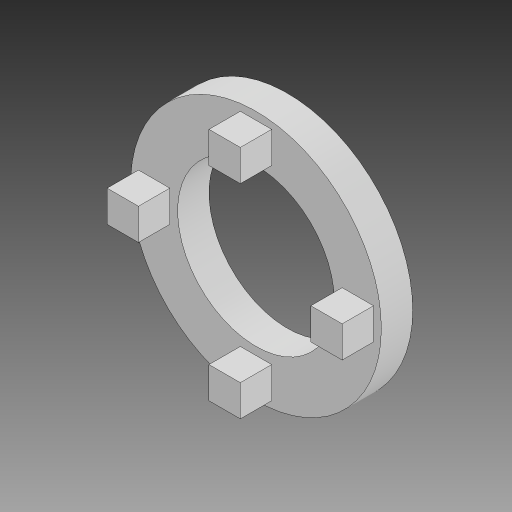
# Autodesk Inventor part: support-ring
Saved by Autodesk Inventor 2023 (Build 270158000, 158)
## iProperties
Created: 2024-01-30
Part Number: support-ring
Material: Všeobecné
Document SubType Name: Modeling
Designer: matej
Mass: 0.0346305 g
Surface Area: 1.18102 cm^2
Volume: 0.0346305 cm^3
Density: 1 g/cm^3
Appearance: Výchozí
Author: matej
Autodesk Inventor part; units mm, degrees
ref_plane "YZ Plane" through (0, 0, 0) normal (1, 0, 0) x (0, 1, 0)
ref_plane "XZ Plane" through (0, 0, 0) normal (0, 1, 0) x (-1, 0, 0)
ref_plane "XY Plane" through (0, 0, 0) normal (0, 0, 1) x (1, 0, 0)
sketch "Náčrt1" plane through (0, 0, 0) normal (0, 0, 1) x (1, 0, 0)
  circle A0 centre (0, 0) radius 2.5
  circle A1 centre (0, 0) radius 4
  dimension "d0" = 5
  dimension "d1" = 8
  constraints: 2 centre point, 2 coincident
  measures "d0" diameter of A0
  measures "d1" diameter of A1
extrude "Vysunutí1" add sketch "Náčrt1" along normal blind 1
sketch "Náčrt2" plane through (0, 0, 1) normal (0, 0, 1) x (1, 0, 0)
  line L0 (-0.5, 3.75) -> (0.5, 3.75)
  line L1 (0.5, 3.75) -> (0.5, 2.75)
  line L2 (0.5, 2.75) -> (-0.5, 2.75)
  line L3 (-0.5, 2.75) -> (-0.5, 3.75)
  line L4 (-0.5, 3.75) -> (0.5, 2.75) construction
  line L5 (0.5, 3.75) -> (-0.5, 2.75) construction
  point P0 (0, 0)
  point P1 (0, 3.25)
  dimension "d4" = 1
  dimension "d5" = 1
  constraints: 12 end point, 2 midpoint, 2 parallel, 1 horizontal, 1 perpendicular
  measures "d4" distance of L1.end L2.end
  measures "d5" distance of L0.end L1.end
extrude "Vysunutí2" add sketch "Náčrt2" along normal blind 1
pattern_circular "Kruhové pole1" count 4 over 360 about axis through (0, 0, 0) along (0, 0, 1) of "Vysunutí2"
